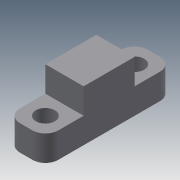
# Autodesk Inventor part: Mirror
Saved by Autodesk Inventor 2015 (Build 190159000, 159)
## iProperties
Created: 2016-11-12
Part Number: Mirror
Material: Generic
Document SubType Name: Modeling
Designer: Aniket Pant
Density: 1 g/cm^3
Appearance: Default
Author: Aniket Pant
Autodesk Inventor part; units mm, degrees
ref_plane "YZ Plane" through (0, 0, 0) normal (1, 0, 0) x (0, 1, 0)
ref_plane "XZ Plane" through (0, 0, 0) normal (0, 1, 0) x (-1, 0, 0)
ref_plane "XY Plane" through (0, 0, 0) normal (0, 0, 1) x (1, 0, 0)
sketch "Sketch2" plane through (0, 0, 0) normal (1, 0, 0) x (0, 1, 0)
  line L0 (28.9006, -29.959) -> (41.6006, -29.959)
  line L1 (41.6006, -29.959) -> (41.6006, -49.009)
  line L2 (41.6006, -49.009) -> (54.3006, -49.009)
  line L3 (54.3006, -49.009) -> (54.3006, -61.709)
  line L4 (54.3006, -61.709) -> (28.9006, -61.709)
  line L5 (28.9006, -61.709) -> (28.9006, -29.959)
  point P0 (0, 0)
  dimension "d0" = 12.7
  dimension "d1" = 19.05
  dimension "d2" = 12.7
  dimension "d3" = 12.7
  constraints: 12 end point, 5 perpendicular, 1 horizontal
  measures "d0" distance of L0.start L0.end
  measures "d1" distance of L0.end L1.end
  measures "d2" distance of L1.end L2.end
  measures "d3" distance of L2.end L3.end
extrude "Extrusion1" add sketch "Sketch2" along normal blind 19.05
sketch "Sketch3" plane through (0, 41.6006, -29.959) normal (0, 1, 0) x (1, 0, 0)
  line L0 (0, 0) -> (0, 19.05) projected
  line L1 (0, 0) -> (19.05, 0) projected
  line L2 (19.05, 19.05) -> (19.05, 0) projected
  line L3 (0, 19.05) -> (19.05, 19.05) projected
  line L4 (0, 19.05) -> (19.05, 19.05) projected
  point P0 (0, -29.959)
  point P1 (9.525, 9.525)
hole "Hole1" at (9.525, 41.6006, -39.484) direction (0, -1, 0) diameter 9.525 end through all
fillet "Fillet1" radius 6.35 2 edges at (19.05, 35.2506, -29.959) (0, 35.2506, -29.959)
mirror "Mirror1" about plane through (0, 28.9006, -61.709) normal (0, 0, -1) of "Hole1", "Extrusion1", "Fillet1"
body "Solid1"
